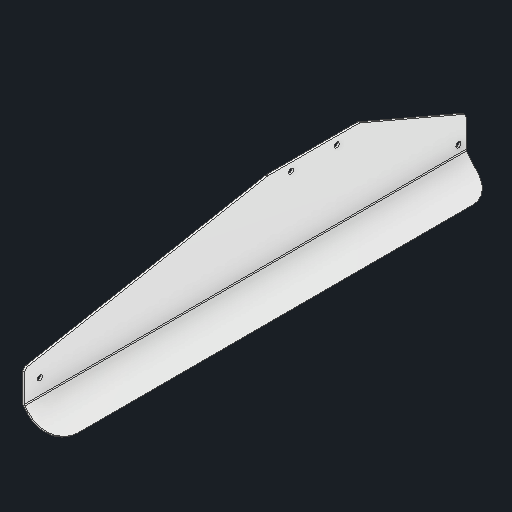
# Autodesk Inventor part: side_panel
Saved by Autodesk Inventor 2025 (Build 290162000, 162)
## iProperties
Created: 2024-07-02
Part Number: side_panel
Material: Acetal Resin, White
Document SubType Name: Modeling
Designer: Averey Ku
Density: 1.425 g/cm^3
Appearance: Smooth - White
Author: Averey Ku
Autodesk Inventor part; units mm, degrees
ref_plane "YZ Plane" through (0, 0, 0) normal (1, 0, 0) x (0, 1, 0)
ref_plane "XZ Plane" through (0, 0, 0) normal (0, 1, 0) x (-1, 0, 0)
ref_plane "XY Plane" through (0, 0, 0) normal (0, 0, 1) x (1, 0, 0)
sketch "main" plane through (0, 0, 0) normal (0, 0, 1) x (1, 0, 0)
  circle A0 centre (51.9329, 240.4167) radius 2.1844
  line L0 (60.6642, 253.1167) -> (43.2017, 253.1167)
  arc A1 (32.8829, 253.1167) -> (7.4829, 227.7167) centre (32.8829, 227.7167) ccw
  line L1 (39.2329, 253.1167) -> (32.8829, 253.1167)
  line L2 (39.2329, 249.9417) -> (39.2329, 253.1167)
  line L3 (39.2329, 253.1167) -> (42.4079, 253.1167)
  line L4 (42.4079, 253.1167) -> (43.2017, 253.1167)
  arc A2 (65.1185, 250.5268) -> (61.9979, 253.1167) centre (61.9979, 249.9417) ccw
  line L5 (61.9979, 253.1167) -> (60.6642, 253.1167)
  line L6 (42.4079, -115.1833) -> (62.5393, -115.1833)
  arc A3 (7.4829, -102.4833) -> (20.1829, -115.1833) centre (20.1829, -102.4833) ccw
  line L7 (20.1829, -115.1833) -> (42.4079, -115.1833)
  arc A4 (62.5393, -115.1833) -> (65.4576, -113.259) centre (62.5393, -112.0083) ccw
  line L8 (39.2329, 249.9417) -> (39.2329, -115.1833)
  line L9 (102.4762, -26.8823) -> (65.4576, -113.259)
  line L10 (102.7329, -25.6316) -> (102.7329, 49.6216)
  line L11 (102.6786, 50.2068) -> (65.1185, 250.5268)
  line L12 (7.4829, 227.7167) -> (7.4829, -102.4833)
  arc A5 (102.7329, 49.6216) -> (102.6786, 50.2068) centre (99.5579, 49.6216) ccw
  circle A6 centre (96.3829, 30.8667) radius 2.1844
  circle A7 centre (96.3829, -7.2333) radius 2.1844
  arc A8 (102.4762, -26.8823) -> (102.7329, -25.6316) centre (99.5579, -25.6316) ccw
  circle A9 centre (45.5829, -108.8333) radius 2.1844
  point P0 (57.0821, 72.2396)
  point P1 (7.4829, 253.1167)
  point P2 (64.6329, -115.1833)
  point P3 (102.7329, -26.2833)
  dimension "d0" = 25.4
  dimension "d1" = 3.175
  dimension "d2" = 3.175
  dimension "d3" = 3.175
  dimension "d4" = 31.75
  dimension "d5" = 90
  dimension "d6" = 25.4
  dimension "d7" = 12.7
  measures "d0" distance of L8.end point (64.633, -115.183)
  measures "d1" radius of A2
  measures "d2" radius of A4
  measures "d3" radius of A5
  measures "d4" distance of L2.end point (7.483, 253.117)
  measures "d5" angle of L12 L1
  measures "d6" radius of A1
  measures "d7" radius of A3
sketch "Sketch1" plane through (0, 0, 0) normal (1, 0, 0) x (0, 1, 0)
  circle A0 centre (6.35, 349.25) radius 2.1844
  line L0 (15.0812, 361.95) -> (-2.3813, 361.95)
  arc A1 (-12.7, 361.95) -> (-38.1, 336.55) centre (-12.7, 336.55) ccw
  line L1 (-6.35, 361.95) -> (-12.7, 361.95)
  line L2 (-6.35, 358.775) -> (-6.35, 361.95)
  line L3 (-6.35, 361.95) -> (-3.175, 361.95)
  line L4 (-3.175, 361.95) -> (-2.3813, 361.95)
  arc A2 (19.5356, 359.3601) -> (16.415, 361.95) centre (16.415, 358.775) ccw
  line L5 (16.415, 361.95) -> (15.0812, 361.95)
  line L6 (-3.175, -6.35) -> (16.9564, -6.35)
  arc A3 (-38.1, 6.35) -> (-25.4, -6.35) centre (-25.4, 6.35) ccw
  line L7 (-25.4, -6.35) -> (-3.175, -6.35)
  arc A4 (16.9564, -6.35) -> (19.8747, -4.4257) centre (16.9564, -3.175) ccw
  line L8 (-6.35, 358.775) -> (-6.35, -6.35)
  line L9 (56.8933, 81.951) -> (19.8747, -4.4257)
  line L10 (57.15, 83.2017) -> (57.15, 158.4549)
  line L11 (57.0956, 159.04) -> (19.5356, 359.3601)
  line L12 (-38.1, 336.55) -> (-38.1, 6.35)
  arc A5 (57.15, 158.4549) -> (57.0956, 159.04) centre (53.975, 158.4549) ccw
  circle A6 centre (50.8, 139.7) radius 2.1844
  circle A7 centre (50.8, 101.6) radius 2.1844
  arc A8 (56.8933, 81.951) -> (57.15, 83.2017) centre (53.975, 83.2017) ccw
  circle A9 centre (0, 0) radius 2.1844
  constraints: 1 other
extrude "Extrusion1" add sketch "Sketch1" along normal blind 1.5875
bend part "Bend Part1" radius 3.175 angle 40 line through (0, -6.35, 358.775) along (0, 0, -1) centre toward (1, 0, 0) moving side (0, -1, 0) both sides no
body "Solid1"
